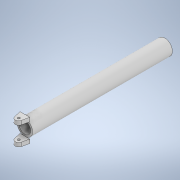
# Autodesk Inventor part: RCT-P004_front_rear_axle_simplified
Saved by Autodesk Inventor 2020 (Build 240168000, 168)
## iProperties
Created: 2019-11-14
Part Number: RCT-P004_front_rear_axle_simplified
Material: Generic
Document SubType Name: Modeling
Designer: maste
Density: 1 g/cm^3
Appearance: Default
Author: maste
Autodesk Inventor part; units mm, degrees
ref_plane "YZ Plane" through (0, 0, 0) normal (1, 0, 0) x (0, 1, 0)
ref_plane "XZ Plane" through (0, 0, 0) normal (0, 1, 0) x (-1, 0, 0)
ref_plane "XY Plane" through (0, 0, 0) normal (0, 0, 1) x (1, 0, 0)
sketch "Sketch1" plane through (0, 0, 0) normal (0, 0, 1) x (1, 0, 0)
  circle A0 centre (0, 0) radius 8
  circle A1 centre (0, 0) radius 6
  dimension "d0" = 16
  dimension "d1" = 12
  constraints: 2 centre point, 2 coincident
  measures "d0" diameter of A0
  measures "d1" diameter of A1
extrude "Extrusion1" add sketch "Sketch1" along normal blind 145
sketch "Sketch2" plane through (0, 0, 145) normal (0, 0, 1) x (1, 0, 0)
  line L0 (-5, 11.75) -> (5, 11.75)
  line L1 (5, 11.75) -> (5, -11.75) construction
  line L2 (5, -11.75) -> (-5, -11.75)
  line L3 (-5, -11.75) -> (-5, 11.75) construction
  line L4 (-5, 7.75) -> (5, 7.75)
  line L5 (-5, -7.75) -> (5, -7.75)
  line L6 (-5, 11.75) -> (-5, 7.75)
  line L7 (5, 11.75) -> (5, 7.75)
  line L8 (-5, -7.75) -> (-5, -11.75)
  line L9 (5, -7.75) -> (5, -11.75)
  point P0 (0, 0)
  dimension "d4" = 23.5
  dimension "d5" = 10
  dimension "d6" = 5
  dimension "d7" = 11.75
  dimension "d8" = 10
  dimension "d9" = 4
  dimension "d10" = 0
  dimension "d11" = 4
  dimension "d12" = 10
  dimension "d13" = 0
  constraints: 20 end point, 3 horizontal, 2 parallel, 1 perpendicular
  measures "d4" distance of L0.end L1.end
  measures "d5" distance of L0.start L0.end
  measures "d6" distance from line of L3 point (0, 0)
  measures "d7" distance from line of L0 point (0, 0)
  measures "d8" distance of L4.start L4.end
  measures "d9" distance between parallel lines of L4 L0
  measures "d10" distance from line of L3 L4.start
  measures "d11" distance between parallel lines of L2 L5
  measures "d12" distance of L5.start L5.end
  measures "d13" distance from line of L1 L5.end
extrude "Extrusion2" add sketch "Sketch2" along normal blind 10
sketch "Sketch3" plane through (-5, 11.75, 145) normal (0, 1, 0) x (1, 0, 0)
  circle A0 centre (5, -6.45) radius 1.25
  line L0 (6.9843, 0) -> (13, 0) projected
  line L1 (11, 0) -> (-1, 0) projected
  circle A1 centre (5, -6.45) radius 3.55
  line L2 (0, 0) -> (0, -10) projected
  line L3 (10, -10) -> (0, -10) projected
  line L4 (10, 0) -> (10, -10) projected
  line L5 (10, 0) -> (8.4725, -7.1879)
  line L6 (0, 0) -> (0, -10) projected
  line L7 (0, 0) -> (1.5275, -7.1879)
  line L8 (0, 0) -> (0, -10)
  line L9 (0, -10) -> (10, -10) projected
  line L10 (0, -10) -> (10, -10)
  line L11 (0, 0) -> (10, 0) projected
  line L12 (10, -10) -> (10, 0)
  point P0 (5, 145)
  point P1 (5, -10)
  dimension "d16" = 2.5
  dimension "d21" = 7.1
  dimension "d22" = 5
  dimension "d23" = 3.55
  constraints: 10 end point, 2 centre point, 2 point on circle, 2 tangent, 1 coincident, 1 collinear, 1 perpendicular, 1 vertical
  measures "d16" diameter of A0
  measures "d21" diameter of A1
  measures "d22" distance from line of L2 A0.centre
  measures "d23" distance from line of L3 A0.centre
extrude "Extrusion3" cut sketch "Sketch3" against normal through all contours A0 | L4 L3 A1 L5 | L7 A1 L3 L2
body "Solid1"
